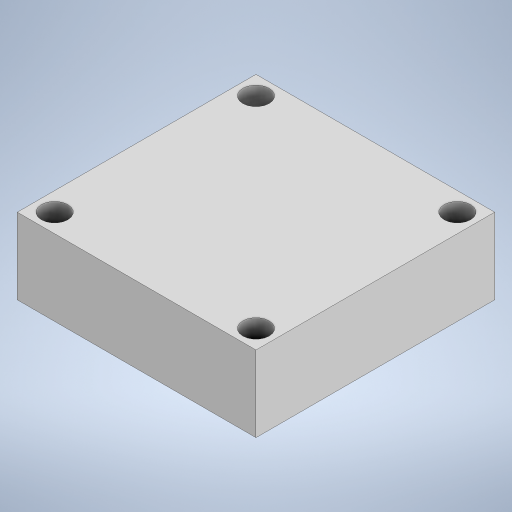
# Autodesk Inventor part: 30x30 stack
Saved by Autodesk Inventor 2023 (Build 270158000, 158)
## iProperties
Created: 2023-01-22
Part Number: 30x30 stack
Material: Generic
Document SubType Name: Modeling
Designer: Steven
Density: 1 g/cm^3
Appearance: Default
Author: Steven
Autodesk Inventor part; units mm, degrees
ref_plane "YZ Plane" through (0, 0, 0) normal (1, 0, 0) x (0, 1, 0)
ref_plane "XZ Plane" through (0, 0, 0) normal (0, 1, 0) x (-1, 0, 0)
ref_plane "XY Plane" through (0, 0, 0) normal (0, 0, 1) x (1, 0, 0)
sketch "Sketch1" plane through (0, 0, 0) normal (0, 1, 0) x (-1, 0, 0)
  line L0 (0, 0) -> (36.15, 0)
  line L1 (36.15, 0) -> (36.15, -36.15)
  line L2 (36.15, -36.15) -> (0, -36.15)
  line L3 (0, -36.15) -> (0, 0)
  dimension "d0" = 36.15
  dimension "d1" = 36.15
  constraints: 8 end point, 2 parallel, 1 horizontal, 1 perpendicular
  measures "d0" distance of L1.end L2.end
  measures "d1" distance of L0.end L1.end
extrude "Extrusion1" add sketch "Sketch1" along normal blind 11.5
sketch "Sketch2" plane through (0, 11.5, 0) normal (0, 1, 0) x (1, 0, 0)
  line L0 (0, 36.15) -> (-36.15, 36.15) construction
  line L1 (-36.15, 36.15) -> (-36.15, 0) construction
  line L2 (-36.15, 0) -> (0, 0) construction
  line L3 (0, 0) -> (0, 36.15) construction
  line L4 (-18.075, 0) -> (-18.075, 36.15) construction
  line L5 (-18.075, 18.075) -> (-33.325, 18.075) construction
  line L6 (-33.325, 18.075) -> (-33.325, 33.325) construction
  circle A0 centre (-33.325, 33.325) radius 2
  circle A1 centre (-33.325, 2.825) radius 2
  circle A2 centre (-2.825, 2.825) radius 2
  circle A3 centre (-2.825, 33.325) radius 2
  dimension "d4" = 15.25
  dimension "d5" = 15.25
  dimension "d6" = 4
  dimension "d9" = 360
  constraints: 6 end point, 4 centre point, 3 midpoint, 1 coincident, 1 horizontal, 1 perpendicular, 9 other
  measures "d4" distance of L5.start L5.end
  measures "d5" distance of L5.end L6.end
  measures "d6" diameter of A0
extrude "Extrusion2" cut sketch "Sketch2" against normal up to surface (11.5 mm away)
body "Solid1"
